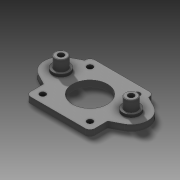
# Autodesk Inventor part: Stepper Atachments
Saved by Autodesk Inventor 2015 (Build 190159000, 159)
## iProperties
Created: 2015-05-08
Part Number: Stepper Atachments
Material: Generic
Document SubType Name: Modeling
Designer: pltwe4
Density: 1 g/cm^3
Appearance: Default
Author: pltwe4
Autodesk Inventor part; units mm, degrees
ref_plane "YZ Plane" through (0, 0, 0) normal (1, 0, 0) x (0, 1, 0)
ref_plane "XZ Plane" through (0, 0, 0) normal (0, 1, 0) x (-1, 0, 0)
ref_plane "XY Plane" through (0, 0, 0) normal (0, 0, 1) x (1, 0, 0)
sketch "Sketch1" plane through (0, 0, 0) normal (0, 0, 1) x (1, 0, 0)
  circle A0 centre (0, 0) radius 11.5
  line L0 (-18, -21) -> (18, -21)
  line L1 (21, -18) -> (21, 18)
  line L2 (18, 21) -> (-18, 21)
  line L3 (-21, 18) -> (-21, -18)
  line L4 (-21, -21) -> (21, 21) construction
  line L5 (21, -21) -> (-21, 21) construction
  circle A1 centre (-15.5, 15.5) radius 1.875
  circle A2 centre (15.5, 15.5) radius 1.875
  circle A3 centre (15.5, -15.5) radius 1.875
  circle A4 centre (-15.5, -15.5) radius 1.875
  line L6 (-15.5, 15.5) -> (15.5, 15.5) construction
  line L7 (15.5, 15.5) -> (15.5, -15.5) construction
  line L8 (15.5, -15.5) -> (-15.5, -15.5) construction
  line L9 (-15.5, 15.5) -> (-15.5, -15.5) construction
  line L10 (-15.5, 15.5) -> (15.5, -15.5) construction
  line L11 (15.5, 15.5) -> (0, 0) construction
  circle A5 centre (-23, 4) radius 3.95
  circle A6 centre (23, 4) radius 3.95
  circle A7 centre (-23, 4) radius 11
  circle A8 centre (23, 4) radius 11
  line L12 (0, 126.4593) -> (0, -125.5407) projected
  line L13 (-111.8366, 0) -> (126.1634, 0) projected
  circle A9 centre (-48.8366, 35.9593) radius 2.0625 projected
  circle A10 centre (-57.8366, 80.4593) radius 2.0625 projected
  circle A11 centre (-66.8366, 35.9593) radius 2.0625 projected
  circle A12 centre (-66.8366, 60.9593) radius 2.0625 projected
  circle A13 centre (-48.8366, 60.9593) radius 2.0625 projected
  circle A14 centre (63.1634, 35.9593) radius 2.0625 projected
  circle A15 centre (72.1634, 80.4593) radius 2.0625 projected
  circle A16 centre (81.1634, 35.9593) radius 2.0625 projected
  circle A17 centre (81.1634, 60.9593) radius 2.0625 projected
  circle A18 centre (63.1634, 60.9593) radius 2.0625 projected
  circle A19 centre (-48.8366, -35.0407) radius 2.0625 projected
  circle A20 centre (-57.8366, -79.5407) radius 2.0625 projected
  circle A21 centre (-66.8366, -35.0407) radius 2.0625 projected
  circle A22 centre (-66.8366, -60.0407) radius 2.0625 projected
  circle A23 centre (-48.8366, -60.0407) radius 2.0625 projected
  circle A24 centre (63.1634, -35.0407) radius 2.0625 projected
  circle A25 centre (63.1634, -60.0407) radius 2.0625 projected
  circle A26 centre (81.1634, -60.0407) radius 2.0625 projected
  circle A27 centre (81.1634, -35.0407) radius 2.0625 projected
  circle A28 centre (72.1634, -79.5407) radius 2.0625 projected
  line L14 (92.1634, -89.5407) -> (92.1634, 90.4593) projected
  line L15 (92.1634, 90.4593) -> (-77.8366, 90.4593) projected
  line L16 (-77.8366, 90.4593) -> (-77.8366, -89.5407) projected
  line L17 (-77.8366, -89.5407) -> (92.1634, -89.5407) projected
  circle A29 centre (-48.8366, 35.9593) radius 2.0625 projected
  circle A30 centre (-57.8366, 80.4593) radius 2.0625 projected
  circle A31 centre (-66.8366, 35.9593) radius 2.0625 projected
  circle A32 centre (-66.8366, 60.9593) radius 2.0625 projected
  circle A33 centre (-48.8366, 60.9593) radius 2.0625 projected
  circle A34 centre (63.1634, 35.9593) radius 2.0625 projected
  circle A35 centre (72.1634, 80.4593) radius 2.0625 projected
  circle A36 centre (81.1634, 35.9593) radius 2.0625 projected
  circle A37 centre (81.1634, 60.9593) radius 2.0625 projected
  circle A38 centre (63.1634, 60.9593) radius 2.0625 projected
  circle A39 centre (-48.8366, -35.0407) radius 2.0625 projected
  circle A40 centre (-57.8366, -79.5407) radius 2.0625 projected
  circle A41 centre (-66.8366, -35.0407) radius 2.0625 projected
  circle A42 centre (-66.8366, -60.0407) radius 2.0625 projected
  circle A43 centre (-48.8366, -60.0407) radius 2.0625 projected
  circle A44 centre (63.1634, -35.0407) radius 2.0625 projected
  circle A45 centre (63.1634, -60.0407) radius 2.0625 projected
  circle A46 centre (81.1634, -60.0407) radius 2.0625 projected
  circle A47 centre (81.1634, -35.0407) radius 2.0625 projected
  circle A48 centre (72.1634, -79.5407) radius 2.0625 projected
  line L18 (92.1634, -89.5407) -> (92.1634, 90.4593) projected
  line L19 (92.1634, 90.4593) -> (-77.8366, 90.4593) projected
  line L20 (-77.8366, 90.4593) -> (-77.8366, -89.5407) projected
  line L21 (-77.8366, -89.5407) -> (92.1634, -89.5407) projected
  arc A49 (-18, 21) -> (-21, 18) centre (-18, 18) ccw
  arc A50 (21, 18) -> (18, 21) centre (18, 18) ccw
  arc A51 (18, -21) -> (21, -18) centre (18, -18) ccw
  arc A52 (-21, -18) -> (-18, -21) centre (-18, -18) ccw
  line L22 (-28.0915, -5.7507) -> (-21, -9.4536)
  line L23 (-28.0915, 13.7507) -> (-21, 17.4536)
  line L24 (28.0915, -5.7507) -> (21, -9.4536)
  line L25 (28.0915, 13.7507) -> (21, 17.4536)
  circle A53 centre (-23, 4) radius 5.5
  circle A54 centre (23, 4) radius 5.5
  dimension "d0" = 23
  dimension "d1" = 3.75
  dimension "d2" = 31
  dimension "d3" = 31
  dimension "d4" = 22
  dimension "d5" = 42
  dimension "d6" = 42
  dimension "d7" = 23
  dimension "d8" = 4
  dimension "d9" = 7.9
  dimension "d10" = 3
  dimension "d11" = 8
  dimension "d12" = 11
  constraints: 32 end point, 15 centre point, 12 point on circle, 12 point on line, 12 tangent, 9 equal radius, 5 coincident, 4 midpoint, 4 perpendicular, 3 equal length, 2 horizontal, 2 parallel, 1 symmetric about line
  measures "d0" diameter of A0
  measures "d1" diameter of A1
  measures "d2" distance of L6.end L6.start
  measures "d3" distance of L7.end L6.end
  measures "d4" diameter of A7
  measures "d5" distance between parallel lines of L0 L2
  measures "d6" distance of L4.end L5.end
  measures "d7" distance from line of A8.centre L12
  measures "d8" distance from line of L13 A6.centre
  measures "d9" diameter of A5
  measures "d10" radius of A49
  measures "d11" distance of L22.start L22.end
  measures "d12" diameter of A53
extrude "Extrusion1" add sketch "Sketch1" along normal blind 4 contours L13 A8 L1 A51 L0 L12 A0 | A0 L12 L2 A50 L1 A8 L13 | A0 L13 A7 L3 A49 L2 L12 | L12 L0 A52 L3 A7 L13 A0 | L13 A54 L1 A8 | A8 L1 A54 L13 | A8 L13 A54 L1 | L1 L25 A8 | A8 L24 L1 | L1 A54 L13 A8 | A54 L1 A6 L13 | L13 L1 A54 | L13 A53 L3 A7 | A7 L3 A53 L13 | A54 L13 L1 A6 | L1 L13 A54 | A7 L13 A53 L3 | L3 L22 A7 | A53 L3 L13 | L13 L3 A5 A53 | A6 L1 | L1 A6 | A53 L13 L3 | A7 L23 L3 | L3 A53 L13 A7 | L13 A53 L3 A5 | A5 L3 | L3 A5
sketch "Sketch2" plane through (0, 0, 4) normal (0, 0, 1) x (1, 0, 0)
  circle A0 centre (0, 0) radius 11.5 projected
  circle A1 centre (-15.5, -15.5) radius 1.875 projected
  circle A2 centre (15.5, -15.5) radius 1.875 projected
  circle A3 centre (15.5, 15.5) radius 1.875 projected
  circle A4 centre (-15.5, 15.5) radius 1.875 projected
  line L0 (28.0915, 13.7507) -> (21, 17.4536) projected
  line L1 (21, 17.4536) -> (21, 18) projected
  arc A5 (21, 18) -> (18, 21) centre (18, 18) ccw projected
  line L2 (18, 21) -> (-18, 21) projected
  arc A6 (-18, 21) -> (-21, 18) centre (-18, 18) ccw projected
  line L3 (-21, 18) -> (-21, 17.4536) projected
  line L4 (-21, 17.4536) -> (-28.0915, 13.7507) projected
  arc A7 (-28.0915, 13.7507) -> (-28.0915, -5.7507) centre (-23, 4) ccw projected
  line L5 (-28.0915, -5.7507) -> (-21, -9.4536) projected
  line L6 (-21, -9.4536) -> (-21, -18) projected
  arc A8 (-21, -18) -> (-18, -21) centre (-18, -18) ccw projected
  line L7 (-18, -21) -> (18, -21) projected
  arc A9 (18, -21) -> (21, -18) centre (18, -18) ccw projected
  line L8 (21, -18) -> (21, -9.4536) projected
  line L9 (21, -9.4536) -> (28.0915, -5.7507) projected
  arc A10 (28.0915, -5.7507) -> (28.0915, 13.7507) centre (23, 4) ccw projected
  circle A11 centre (23, 4) radius 5.5
  circle A12 centre (-23, 4) radius 5.5
  circle A13 centre (23, 4) radius 3.95
  circle A14 centre (-23, 4) radius 3.95
  dimension "d15" = 11
  dimension "d16" = 7.9
  dimension "d17" = 7.9
  dimension "d18" = 11
  constraints: 4 centre point, 4 coincident
  measures "d15" diameter of A11
  measures "d16" diameter of A13
  measures "d17" diameter of A14
  measures "d18" diameter of A12
extrude "Extrusion2" add sketch "Sketch2" along normal blind 8.75 contours A13 | A14
extrude "Extrusion3" add sketch "Sketch2" along normal blind 1.75 contours A11 | A12
fillet "Fillet1" radius 0.5 2 edges at (19.05, 4, 12.75) (-26.95, 4, 12.75)
sketch "Sketch3" plane through (23, 4, 12.75) normal (0, 0, 1) x (1, 0, 0)
  circle A0 centre (0, 0) radius 3.45 projected
  circle A1 centre (-46, 0) radius 3.45 projected
  circle A2 centre (0, 0) radius 1.925
  circle A3 centre (-46, 0) radius 1.925
  point P0 (-23, -4)
  dimension "d24" = 3.85
  constraints: 2 centre point, 2 coincident, 1 equal radius
  measures "d24" diameter of A2
extrude "Extrusion4" cut sketch "Sketch3" against normal blind 8 contours A2 | A3
body "Solid1"
